Autodesk Inventor part; units mm, degrees
(part 2 of 2)
extrude "Cut10" cut sketch "Sketch17" against normal blind 1.5875 contours A302 L31 | L31 A302 L213 A303 L214 | A300 L31 | L31 A300 L211 A301 L212 | A298 L209 A299 L32 E1 L31 | L31 E1 L32 A299 L210 A298 | L234 A322 L233 L33 | L33 L233 L26 L234 | L26 L233 A323 L234 | L232 A320 L231 L33 | L33 L231 L26 L232 | L26 L231 A321 L232 | L247 A337 L248 L37 | L37 L248 A336 L247 | A332 L243 A333 L43 | L43 A333 L244 A332 | A330 L241 A331 L45 | L45 A331 L242 A330 | A201 L112 A200 L51 | L51 A200 L111 A201 | A181 L92 A180 L51 | L51 A180 L91 A181 | A186 L97 A187 L52 | L52 A187 L98 A186 | A206 L117 A207 L52 | L52 A207 L118 A206 | L76 A164 L75 L54 | L54 L75 A165 L76 | L74 A162 L73 L54 | L54 L73 A163 L74 | A155 L66 A154 L65 | A173 L84 A172 L83 | A175 L86 A174 L85 | A183 L94 A182 L93 | A185 L96 A184 L95 | A193 L104 A192 L103 | A195 L106 A194 L105 | A203 L114 A202 L113 | A205 L116 A204 L115 | A213 L124 A212 L123 | A215 L126 A214 L125 | A223 L134 A222 L133 | A225 L136 A224 L135 | A233 L144 A232 L143 | A243 L154 A242 L153 | A245 L156 A244 L155 | A263 L174 A262 L173 | A265 L176 A264 L175 | A283 L194 A282 L193 | A285 L196 A284 L195 | A295 L206 A294 L205 | A309 L220 A308 L219 | A315 L226 A314 L225 | A329 L240 A328 L239 | A335 L246 A334 L245 | A339 L250 A338 L249 | A341 L252 A340 L251 | A343 L254 A342 L253 | A345 L256 A344 L255 | A347 L258 A346 L257 | A349 L260 A348 L259
equation "\"d17\" = Thickness"
equation "\"d65\" = Thickness"
equation "\"BendRadius\" = Thickness"
equation "\"BendReliefWidth\" = Thickness"
equation "\"BendReliefDepth\" = 0.5 * Thickness"
equation "\"CornerReliefSize\" = 4 * Thickness"
equation "\"MinimumRemnant\" = 2 * Thickness"
equation "\"TransitionRadius\" = BendRadius"
equation "\"JacobiRadiusSize\" = Thickness"
equation "\"GapSize\" = Thickness"
equation "\"d2\" = BendRadius"
equation "\"Thickness\" = 1.5875"
body "Solid1"
